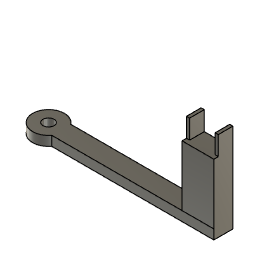
BOTON_BASE2 (Autodesk Fusion 360 design; units mm, degrees)
Autodesk Fusion 360 part; units mm, degrees
sketch "Sketch1" plane through (0, 0, 0) normal (0, 0, 1) x (1, 0, 0)
  line L0 (55, -3) -> (4, -3)
  line L1 (-55, -3) -> (-55, 3)
  line L2 (4, 3) -> (55, 3)
  line L3 (55, 3) -> (55, -3)
  arc A0 (4, 3) -> (4, -3) centre (0, 0) ccw
  dimension "d1" = 10
  dimension "d3" = 6
  constraint horizontal L0
  constraint perpendicular L0 L1
  constraint parallel L0 L2
  constraint parallel L1 L3
  constraint coincident A0.centre origin
  measures "d1" diameter of A0
  measures "d3" distance of L1.start L1.end
extrude "Extrude1" add sketch "Sketch1" along normal blind 3
sketch "Sketch2" plane through (0, 0, 3) normal (0, 0, 1) x (-1, 0, 0)
  line L0 (-55, -3) -> (-4, -3)
  arc A0 (-4, -3) -> (-4, 3) centre (0, 0) ccw
  line L1 (-4, 3) -> (-55, 3)
  line L2 (-55, 3) -> (-55, -3)
  circle A1 centre (0, 0) radius 1.75
  dimension "d8" = 3.5
  constraint coincident A0.centre A1.centre
  measures "d8" diameter of A1
extrude "Extrude2" cut sketch "Sketch2" against normal blind 3 contours A1
sketch "Sketch3" plane through (0, 0, 3) normal (0, 0, 1) x (-1, 0, 0)
  circle A0 centre (0, 0) radius 1.75
  line L0 (-55, -3) -> (-4, -3)
  arc A1 (-4, -3) -> (-4, 3) centre (0, 0) ccw
  line L1 (-4, 3) -> (-55, 3)
  line L2 (-55, 3) -> (-55, -3)
  line L3 (-55, -3) -> (-45, -3)
  line L4 (-45, -3) -> (-45, 3)
  line L5 (-45, 3) -> (-55, 3)
  line L6 (-55, 3) -> (-55, -3)
  dimension "d11" = 10
  constraint horizontal L3
  constraint vertical L4
  constraint horizontal L5
  constraint vertical L6
  constraint coincident L1 L4.end
  constraint coincident L0.start L2.end
  measures "d11" distance of L0.start L3.end
extrude "Extrude3" add sketch "Sketch3" along normal blind 25 contours L0 L1 L2 L3 L4 L5 L6
sketch "Sketch4" plane through (0, 0, 28) normal (0, 0, 1) x (-1, 0, 0)
  line L0 (-55, 3) -> (-55, -3)
  line L1 (-55, -3) -> (-45, -3)
  line L2 (-45, -3) -> (-45, 3)
  line L3 (-45, 3) -> (-55, 3)
  line L4 (-45, -3) -> (-46, -3)
  line L5 (-46, -3) -> (-46, 1.6)
  line L6 (-46, 1.6) -> (-45, 1.6)
  line L7 (-45, 1.6) -> (-45, -3)
  line L8 (-55, -3) -> (-54, -3)
  line L9 (-54, -3) -> (-54, 1.6)
  line L10 (-54, 1.6) -> (-55, 1.6)
  line L11 (-55, 1.6) -> (-55, -3)
  dimension "d14" = 4.6
  dimension "d15" = 1
  constraint horizontal L4
  constraint vertical L5
  constraint horizontal L6
  constraint vertical L7
  constraint coincident L1.end L2.start
  constraint horizontal L8
  constraint vertical L9
  constraint horizontal L10
  constraint vertical L11
  constraint coincident L0.end L1.start
  constraint equal L7 L11
  constraint equal L4 L8
  measures "d14" distance of L0.end L10.end
  measures "d15" distance of L0.end L8.end
extrude "Extrude4" cut sketch "Sketch4" against normal blind 6 contours L0 L1 L2 L3 L5 L6 L9 L10
